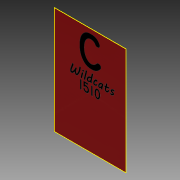
# Autodesk Inventor part: banner1
Saved by Autodesk Inventor 2014 (Build 180170000, 170)
## iProperties
Created: 2015-04-10
Part Number: banner1
Material: Generic
Document SubType Name: Modeling
Designer: Gus
Density: 1 g/cm^3
Appearance: 4in Square - Light Blue
Author: Gus
Autodesk Inventor part; units mm, degrees
ref_plane "YZ Plane" through (0, 0, 0) normal (1, 0, 0) x (0, 1, 0)
ref_plane "XZ Plane" through (0, 0, 0) normal (0, 1, 0) x (-1, 0, 0)
ref_plane "XY Plane" through (0, 0, 0) normal (0, 0, 1) x (1, 0, 0)
sketch "Sketch1" plane through (0, 0, 0) normal (0, 0, 1) x (1, 0, 0)
  line L0 (0, 0) -> (609.6, 0)
  line L1 (609.6, 0) -> (609.6, 914.4)
  line L2 (609.6, 914.4) -> (0, 914.4)
  line L3 (0, 914.4) -> (0, 0)
  dimension "d0" = 609.6
  dimension "d1" = 914.4
  constraints: 8 end point, 2 parallel, 1 horizontal, 1 perpendicular
  measures "d0" distance of L2.end L1.end
  measures "d1" distance of L1.end L0.end
extrude "Extrusion1" add sketch "Sketch1" along normal blind 0.254
sketch "Sketch2" plane through (0, 0, 0.254) normal (0, 0, 1) x (1, 0, 0)
  line L0 (0, 0) -> (609.6, 0) projected
  line L1 (609.6, 0) -> (609.6, 914.4) projected
  line L2 (609.6, 914.4) -> (0, 914.4) projected
  line L3 (0, 914.4) -> (0, 0) projected
  line L4 (125.4958, 588.6079) -> (509.7299, 588.6079) construction
  line L5 (509.7299, 588.6079) -> (509.7299, 339.0137) construction
  line L6 (509.7299, 339.0137) -> (125.4958, 339.0137) construction
  line L7 (125.4958, 339.0137) -> (125.4958, 588.6079) construction
  line L8 (199.1824, 873.5297) -> (311.9747, 873.5297) construction
  line L9 (311.9747, 873.5297) -> (311.9747, 744.8866) construction
  line L10 (311.9747, 744.8866) -> (199.1824, 744.8866) construction
  line L11 (199.1824, 744.8866) -> (199.1824, 873.5297) construction
  constraints: 4 other
body "Solid1"
